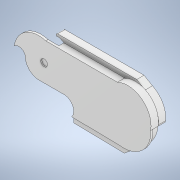
# Autodesk Inventor part: Pieza4
Saved by Autodesk Inventor 2022 (Build 260153000, 153)
## iProperties
Created: 2022-11-04
Part Number: Pieza4
Material: Resina acetálica, blanca
Document SubType Name: Modeling
Designer: Mauricio Guerrero
Density: 1.425 g/cm^3
Appearance: Suave - Blanco
Author: Mauricio Guerrero
Autodesk Inventor part; units mm, degrees
ref_plane "YZ Plane" through (0, 0, 0) normal (1, 0, 0) x (0, 1, 0)
ref_plane "XZ Plane" through (0, 0, 0) normal (0, 1, 0) x (-1, 0, 0)
ref_plane "XY Plane" through (0, 0, 0) normal (0, 0, 1) x (1, 0, 0)
sketch "Boceto1" plane through (0, 0, 0) normal (0, 0, 1) x (1, 0, 0)
  line L0 (26.0808, -19.0043) -> (25.4762, -18.9788)
  line L1 (8.8579, -18.68) -> (25.4762, -18.9788)
  line L2 (0, 0.0061) -> (25.0257, 0.0061)
  line L3 (0, 0.0061) -> (25.0257, 0.0061)
  line L4 (-1.5746, -5.9665) -> (-0.3149, -5.9665)
  circle A0 centre (-0.9088, -7.0094) radius 1.2002
  arc A1 (25.9493, -18.9873) -> (36.7928, -8.9256) centre (27.2383, -9.5026) ccw
  line L5 (37.0197, -12.6823) -> (36.7928, -8.9256) construction
  line L6 (5.8136, -13.2096) -> (-2.0458, -13.2096)
  arc A2 (8.8579, -18.68) -> (5.8136, -13.2096) centre (6.1366, -16.6121) ccw
  arc A3 (-7.6246, -8.019) -> (-2.0458, -13.2096) centre (-2.6389, -8.2538) ccw
  line L7 (-7.6246, -8.019) -> (-7.6206, -7.9467)
  arc A4 (-7.6246, -8.019) -> (-11.4954, -7.0855) centre (-9.8812, -8.8845) ccw
  arc A5 (-0.3158, 0.0061) -> (-11.4954, -7.0855) centre (-2.8556, -8.3478) ccw
  line L8 (-0.3158, 0.0061) -> (0, 0.0061)
  arc A6 (36.7928, -8.9256) -> (25.0257, 0.0061) centre (28.6695, -7.4106) ccw
  point P0 (0, 0)
  dimension "d4" = 6.2002
  constraints: 18 end point, 14 point on circle, 6 centre point, 3 horizontal, 1 point on line, 1 tangent, 3 other
  measures "d4" distance from line of L6 point (-0.909, -7.009)
extrude "Extrusión1" add sketch "Boceto1" along normal blind 0.8
sketch "Boceto2" plane through (0, 0, 0) normal (0, 0, -1) x (-1, 0, 0)
  arc A0 (-3.4903, 0.0061) -> (-8.8579, -18.68) centre (12.417, -14.6773) ccw
  line L0 (-3.4903, 0.0061) -> (-25.0257, 0.0061)
  arc A1 (-25.0257, 0.0061) -> (-36.7928, -8.9256) centre (-28.6695, -7.4106) ccw projected
  arc A2 (-25.0257, 0.0061) -> (-36.7928, -8.9256) centre (-28.6695, -7.4106) ccw
  arc A3 (-36.7928, -8.9256) -> (-32.6377, -16.5472) centre (-25.6771, -7.8089) ccw
  line L1 (-32.6377, -16.5472) -> (-26.6305, -21.3323)
  line L2 (-26.6305, -21.3323) -> (-8.816, -21.0119)
  line L3 (-8.816, -21.0119) -> (-8.8579, -18.68)
  point P0 (0, 0)
  point P1 (-25.4762, -18.9788)
  point P2 (-27.1681, -7.0263)
  point P3 (-11.7669, -7.0263)
  constraints: 8 end point, 6 point on circle, 3 centre point, 1 concentric, 1 horizontal, 1 perpendicular
extrude "Extrusión2" add sketch "Boceto2" along normal blind 1.8
sketch "Boceto3" plane through (0, 0, -1.8) normal (0, 0, -1) x (-1, 0, 0)
  arc A0 (-32.2242, -0.1005) -> (-36.8492, -8.491) centre (-28.759, -7.4805) ccw
  line L0 (-36.7928, -8.9256) -> (-36.0178, -9.1355)
  arc A1 (-25.0257, -0.6131) -> (-36.0178, -9.1355) centre (-28.5733, -7.3874) ccw
  line L1 (-25.0257, -0.6131) -> (-4.5645, -0.6131)
  line L2 (-4.5645, -0.6131) -> (-3.551, -0.0288)
  line L3 (-3.4274, 0.0367) -> (-2.3154, 0.578)
  line L4 (-1.901, 1.6527) -> (-29.2586, 1.6527)
  line L5 (-29.2586, 1.6527) -> (-33.0913, -0.6131)
  line L6 (-36.8492, -8.491) -> (-36.7928, -8.9256)
  line L7 (-1.4401, 0.7797) -> (-0.839, 0.7797)
  line L8 (-0.839, 0.7797) -> (-0.7783, 1.0384)
  line L9 (-1.265, 1.6527) -> (-3.3088, 1.6527)
  arc A2 (-3.4274, 0.0367) -> (-3.551, -0.0288) centre (-2.5521, -1.7616) ccw
  arc A3 (-1.4401, 0.7797) -> (-2.3154, 0.578) centre (-1.4401, -1.2203) ccw
  arc A4 (-0.7783, 1.0384) -> (-1.265, 1.6527) centre (-1.265, 1.1527) ccw
  point P0 (-3.4903, 0.0061)
  point P1 (-26.0808, -19.0043)
  point P2 (-8.8579, -18.68)
  point P3 (-1.901, 0.7797)
  point P4 (-36.5961, -8.5348)
  point P5 (-33.0913, -0.6131)
  dimension "d15" = 2
  dimension "d16" = 0.5
  constraints: 20 end point, 10 point on circle, 6 tangent, 5 centre point, 5 point on line, 3 horizontal, 1 equal radius
  measures "d15" radius of A2
  measures "d16" radius of A4
extrude "Extrusión3" add sketch "Boceto3" along normal blind 2.6
sketch "Boceto4" plane through (0, 0, 0) normal (0, 0, -1) x (-1, 0, 0)
  circle A0 centre (0.9088, -7.0094) radius 1.2002 projected
  circle A1 centre (0.9088, -7.0094) radius 1.2002
  point P0 (0, 0)
  constraints: 1 centre point, 1 coincident
extrude "Extrusión4" add sketch "Boceto4" along normal blind 1
sketch "Boceto5" plane through (-0.9088, -7.0094, 0) normal (0, 0, 1) x (1, 0, 0)
  circle A0 centre (0, 0) radius 1.2002 projected
  circle A1 centre (0, 0) radius 1.2002
  point P0 (0.9088, 7.0094)
  constraints: 1 centre point, 1 coincident
extrude "Extrusión5" add sketch "Boceto5" along normal blind 0.4
